Autodesk Inventor part; units mm, degrees
(part 2 of 2)
sketch "Sketch7" plane through (0, 0, 0) normal (0, -1, 0) x (1, 0, 0)
  line L0 (19.8255, 40.6005) -> (19.4339, 40.6005)
  line L1 (19.4339, 40.6005) -> (19.4339, 41.8395)
  line L2 (19.4339, 41.8395) -> (19.8255, 41.8395)
  line L3 (19.8255, 41.8395) -> (19.8255, 40.6005)
  line L4 (34.3949, 40.6005) -> (34.0033, 40.6005)
  line L5 (34.0033, 40.6005) -> (34.0033, 41.8395)
  line L6 (34.0033, 41.8395) -> (34.3949, 41.8395)
  line L7 (34.3949, 41.8395) -> (34.3949, 40.6005)
  line L8 (23.0894, 38.36) -> (23.0894, 38.66)
  line L9 (23.0894, 38.66) -> (23.7394, 38.66)
  line L10 (23.7394, 38.66) -> (23.7394, 38.36)
  line L11 (23.7394, 38.36) -> (23.0894, 38.36)
  line L12 (26.2394, 38.36) -> (25.5894, 38.36)
  line L13 (25.5894, 38.36) -> (25.5894, 38.66)
  line L14 (25.5894, 38.66) -> (26.2394, 38.66)
  line L15 (26.2394, 38.66) -> (26.2394, 38.36)
  line L16 (30.7394, 38.66) -> (30.7394, 38.36)
  line L17 (30.7394, 38.36) -> (30.0894, 38.36)
  line L18 (30.0894, 38.36) -> (30.0894, 38.66)
  line L19 (30.0894, 38.66) -> (30.7394, 38.66)
  line L20 (28.2394, 38.36) -> (27.5894, 38.36)
  line L21 (27.5894, 38.36) -> (27.5894, 38.66)
  line L22 (27.5894, 38.66) -> (28.2394, 38.66)
  line L23 (28.2394, 38.66) -> (28.2394, 38.36)
  line L24 (7.6945, 42.75) -> (6.6945, 42.75)
  line L25 (6.6945, 42.75) -> (6.6945, 43.25)
  line L26 (6.6945, 43.25) -> (7.6945, 43.25)
  line L27 (7.6945, 43.25) -> (7.6945, 42.75)
  line L28 (4.9445, 38.5) -> (4.9445, 37.5)
  line L29 (4.9445, 37.5) -> (4.4445, 37.5)
  line L30 (4.4445, 37.5) -> (4.4445, 38.5)
  line L31 (4.4445, 38.5) -> (4.9445, 38.5)
  line L32 (9.9445, 38.5) -> (9.9445, 37.5)
  line L33 (9.9445, 37.5) -> (9.4445, 37.5)
  line L34 (9.4445, 37.5) -> (9.4445, 38.5)
  line L35 (9.4445, 38.5) -> (9.9445, 38.5)
  line L36 (2.4445, 38.5) -> (2.4445, 37.5)
  line L37 (2.4445, 37.5) -> (1.9445, 37.5)
  line L38 (1.9445, 37.5) -> (1.9445, 38.5)
  line L39 (1.9445, 38.5) -> (2.4445, 38.5)
  line L40 (12.4445, 38.5) -> (12.4445, 37.5)
  line L41 (12.4445, 37.5) -> (11.9445, 37.5)
  line L42 (11.9445, 37.5) -> (11.9445, 38.5)
  line L43 (11.9445, 38.5) -> (12.4445, 38.5)
  line L44 (-20.3177, 45.8349) -> (-20.3177, 46.9651)
  line L45 (-20.3177, 46.9651) -> (-20.0677, 46.9651)
  line L46 (-20.0677, 46.9651) -> (-20.0677, 45.8349)
  line L47 (-20.0677, 45.8349) -> (-20.3177, 45.8349)
  line L48 (-5.2277, 42.75) -> (-5.2277, 42.5754)
  arc A0 (-8.0277, 42.5754) -> (-5.2277, 42.5754) centre (-6.6277, 43.35) ccw
  line L49 (-8.0277, 42.5754) -> (-8.0277, 43.2)
  line L50 (-8.0277, 43.2) -> (-7.3277, 43.2)
  line L51 (-7.3277, 43.2) -> (-7.3277, 42.75)
  line L52 (-7.3277, 42.75) -> (-5.2277, 42.75)
  line L53 (-5.2277, 44.1246) -> (-5.2277, 43.95)
  line L54 (-5.2277, 43.95) -> (-7.3277, 43.95)
  line L55 (-7.3277, 43.95) -> (-7.3277, 43.5)
  line L56 (-7.3277, 43.5) -> (-8.0277, 43.5)
  line L57 (-8.0277, 43.5) -> (-8.0277, 44.1246)
  arc A1 (-5.2277, 44.1246) -> (-8.0277, 44.1246) centre (-6.6277, 43.35) ccw
  arc A2 (-19.4577, 42.5754) -> (-16.6577, 42.5754) centre (-18.0577, 43.35) ccw
  line L58 (-19.4577, 42.5754) -> (-19.4577, 42.75)
  line L59 (-19.4577, 42.75) -> (-17.3577, 42.75)
  line L60 (-17.3577, 42.75) -> (-17.3577, 43.2)
  line L61 (-17.3577, 43.2) -> (-16.6577, 43.2)
  line L62 (-16.6577, 43.2) -> (-16.6577, 42.5754)
  arc A3 (-16.6577, 44.1246) -> (-19.4577, 44.1246) centre (-18.0577, 43.35) ccw
  line L63 (-16.6577, 44.1246) -> (-16.6577, 43.5)
  line L64 (-16.6577, 43.5) -> (-17.3577, 43.5)
  line L65 (-17.3577, 43.5) -> (-17.3577, 43.95)
  line L66 (-17.3577, 43.95) -> (-19.4577, 43.95)
  line L67 (-19.4577, 43.95) -> (-19.4577, 44.1246)
  arc A4 (-16.7877, 37.215) -> (-16.7877, 36.765) centre (-16.7877, 36.99) ccw
  arc A5 (-16.7877, 36.765) -> (-16.7877, 37.215) centre (-16.7877, 36.99) ccw
  arc A6 (-14.2477, 37.215) -> (-14.2477, 36.765) centre (-14.2477, 36.99) ccw
  arc A7 (-14.2477, 36.765) -> (-14.2477, 37.215) centre (-14.2477, 36.99) ccw
  arc A8 (-11.7077, 37.215) -> (-11.7077, 36.765) centre (-11.7077, 36.99) ccw
  arc A9 (-11.7077, 36.765) -> (-11.7077, 37.215) centre (-11.7077, 36.99) ccw
  arc A10 (-9.1677, 37.215) -> (-9.1677, 36.765) centre (-9.1677, 36.99) ccw
  arc A11 (-9.1677, 36.765) -> (-9.1677, 37.215) centre (-9.1677, 36.99) ccw
  arc A12 (-15.5177, 34.675) -> (-15.5177, 34.225) centre (-15.5177, 34.45) ccw
  arc A13 (-15.5177, 34.225) -> (-15.5177, 34.675) centre (-15.5177, 34.45) ccw
  arc A14 (-12.9777, 34.675) -> (-12.9777, 34.225) centre (-12.9777, 34.45) ccw
  arc A15 (-12.9777, 34.225) -> (-12.9777, 34.675) centre (-12.9777, 34.45) ccw
  arc A16 (-10.4377, 34.675) -> (-10.4377, 34.225) centre (-10.4377, 34.45) ccw
  arc A17 (-10.4377, 34.225) -> (-10.4377, 34.675) centre (-10.4377, 34.45) ccw
  arc A18 (-7.8977, 34.675) -> (-7.8977, 34.225) centre (-7.8977, 34.45) ccw
  arc A19 (-7.8977, 34.225) -> (-7.8977, 34.675) centre (-7.8977, 34.45) ccw
  line L68 (-4.6177, 45.8349) -> (-4.6177, 46.9651)
  line L69 (-4.6177, 46.9651) -> (-4.3677, 46.9651)
  line L70 (-4.3677, 46.9651) -> (-4.3677, 45.8349)
  line L71 (-4.3677, 45.8349) -> (-4.6177, 45.8349)
  line L72 (-30.7746, 41.22) -> (-30.7746, 41.78)
  arc A20 (-30.7746, 41.7814) -> (-30.7746, 41.78) centre (-30.5546, 41.78) ccw
  arc A21 (-30.5546, 42) -> (-30.7746, 41.7814) centre (-30.5546, 41.78) ccw
  line L73 (-30.5546, 42) -> (-29.9946, 42)
  arc A22 (-29.9919, 42) -> (-29.9946, 42) centre (-29.9946, 41.78) ccw
  arc A23 (-29.7746, 41.78) -> (-29.9919, 42) centre (-29.9946, 41.78) ccw
  line L74 (-29.7746, 41.78) -> (-29.7746, 41.22)
  arc A24 (-29.7746, 41.2186) -> (-29.7746, 41.22) centre (-29.9946, 41.22) ccw
  arc A25 (-29.9946, 41) -> (-29.7746, 41.2186) centre (-29.9946, 41.22) ccw
  line L75 (-29.9946, 41) -> (-30.5546, 41)
  arc A26 (-30.7746, 41.2186) -> (-30.5546, 41) centre (-30.5546, 41.22) ccw
  arc A27 (-30.7746, 41.22) -> (-30.7746, 41.2186) centre (-30.5546, 41.22) ccw
  line L76 (-25.7746, 41.22) -> (-25.7746, 41.78)
  arc A28 (-25.7746, 41.7814) -> (-25.7746, 41.78) centre (-25.5546, 41.78) ccw
  arc A29 (-25.5546, 42) -> (-25.7746, 41.7814) centre (-25.5546, 41.78) ccw
  line L77 (-25.5546, 42) -> (-24.9946, 42)
  arc A30 (-24.9919, 42) -> (-24.9946, 42) centre (-24.9946, 41.78) ccw
  arc A31 (-24.7746, 41.78) -> (-24.9919, 42) centre (-24.9946, 41.78) ccw
  line L78 (-24.7746, 41.78) -> (-24.7746, 41.22)
  arc A32 (-24.7746, 41.2186) -> (-24.7746, 41.22) centre (-24.9946, 41.22) ccw
  arc A33 (-24.9946, 41) -> (-24.7746, 41.2186) centre (-24.9946, 41.22) ccw
  line L79 (-24.9946, 41) -> (-25.5546, 41)
  arc A34 (-25.7746, 41.2186) -> (-25.5546, 41) centre (-25.5546, 41.22) ccw
  arc A35 (-25.7746, 41.22) -> (-25.7746, 41.2186) centre (-25.5546, 41.22) ccw
  line L80 (-33.125, 30.2845) -> (-32.455, 30.2845)
  line L81 (-32.455, 30.2845) -> (-32.455, 29.6145)
  line L82 (-32.455, 29.6145) -> (-33.125, 29.6145)
  line L83 (-33.125, 29.6145) -> (-33.125, 30.2845)
  line L84 (-33.125, 27.7445) -> (-32.455, 27.7445)
  line L85 (-32.455, 27.7445) -> (-32.455, 27.0745)
  line L86 (-32.455, 27.0745) -> (-33.125, 27.0745)
  line L87 (-33.125, 27.0745) -> (-33.125, 27.7445)
  circle A36 centre (31.5, -29) radius 2.1 projected
  circle A37 centre (-25.5, 29) radius 2.1 projected
  circle A38 centre (-25.5, -29) radius 2.1 projected
  circle A39 centre (31.5, 29) radius 2.1 projected
  arc A40 (40.5, -27.5) -> (36.5, -31.5) centre (40.5, -31.5) ccw projected
  line L88 (36.5, -31.5) -> (36.5, -44.5) projected
  arc A41 (33.5, -47.5) -> (36.5, -44.5) centre (33.5, -44.5) ccw projected
  line L89 (33.5, -47.5) -> (-33.5, -47.5) projected
  arc A42 (-36.5, -44.5) -> (-33.5, -47.5) centre (-33.5, -44.5) ccw projected
  line L90 (-36.5, -44.5) -> (-36.5, -31.5) projected
  arc A43 (-36.5, -31.5) -> (-40.5, -27.5) centre (-40.5, -31.5) ccw projected
  line L91 (-40.5, -27.5) -> (-44.5, -27.5) projected
  arc A44 (-47.5, -24.5) -> (-44.5, -27.5) centre (-44.5, -24.5) ccw projected
  line L92 (-47.5, -24.5) -> (-47.5, 24.5) projected
  arc A45 (-44.5, 27.5) -> (-47.5, 24.5) centre (-44.5, 24.5) ccw projected
  line L93 (-44.5, 27.5) -> (-40.5, 27.5) projected
  arc A46 (-40.5, 27.5) -> (-36.5, 31.5) centre (-40.5, 31.5) ccw projected
  line L94 (-36.5, 31.5) -> (-36.5, 44.5) projected
  arc A47 (-33.5, 47.5) -> (-36.5, 44.5) centre (-33.5, 44.5) ccw projected
  line L95 (-33.5, 47.5) -> (33.5, 47.5) projected
  arc A48 (36.5, 44.5) -> (33.5, 47.5) centre (33.5, 44.5) ccw projected
  line L96 (36.5, 44.5) -> (36.5, 31.5) projected
  arc A49 (36.5, 31.5) -> (40.5, 27.5) centre (40.5, 31.5) ccw projected
  line L97 (40.5, 27.5) -> (44.5, 27.5) projected
  arc A50 (47.5, 24.5) -> (44.5, 27.5) centre (44.5, 24.5) ccw projected
  line L98 (47.5, 24.5) -> (47.5, -24.5) projected
  arc A51 (44.5, -27.5) -> (47.5, -24.5) centre (44.5, -24.5) ccw projected
  line L99 (44.5, -27.5) -> (40.5, -27.5) projected
  circle A52 centre (40.395, 20.471) radius 1.5 projected
  circle A53 centre (-40.395, 20.471) radius 1.5 projected
  circle A54 centre (40.395, -20.471) radius 1.5 projected
  line L100 (43.9275, -13.9528) -> (44.5975, -13.9528)
  line L101 (44.5975, -13.9528) -> (44.5975, -14.6228)
  line L102 (44.5975, -14.6228) -> (43.9275, -14.6228)
  line L103 (43.9275, -14.6228) -> (43.9275, -13.9528)
  line L104 (43.9275, -11.4128) -> (44.5975, -11.4128)
  line L105 (44.5975, -11.4128) -> (44.5975, -12.0828)
  line L106 (44.5975, -12.0828) -> (43.9275, -12.0828)
  line L107 (43.9275, -12.0828) -> (43.9275, -11.4128)
  line L108 (43.9275, -8.8728) -> (44.5975, -8.8728)
  line L109 (44.5975, -8.8728) -> (44.5975, -9.5428)
  line L110 (44.5975, -9.5428) -> (43.9275, -9.5428)
  line L111 (43.9275, -9.5428) -> (43.9275, -8.8728)
  line L112 (43.9275, -6.3328) -> (44.5975, -6.3328)
  line L113 (44.5975, -6.3328) -> (44.5975, -7.0028)
  line L114 (44.5975, -7.0028) -> (43.9275, -7.0028)
  line L115 (43.9275, -7.0028) -> (43.9275, -6.3328)
  line L116 (43.9275, -3.7928) -> (44.5975, -3.7928)
  line L117 (44.5975, -3.7928) -> (44.5975, -4.4628)
  line L118 (44.5975, -4.4628) -> (43.9275, -4.4628)
  line L119 (43.9275, -4.4628) -> (43.9275, -3.7928)
  line L120 (43.9275, -1.2528) -> (44.5975, -1.2528)
  line L121 (44.5975, -1.2528) -> (44.5975, -1.9228)
  line L122 (44.5975, -1.9228) -> (43.9275, -1.9228)
  line L123 (43.9275, -1.9228) -> (43.9275, -1.2528)
  line L124 (43.9275, 1.2872) -> (44.5975, 1.2872)
  line L125 (44.5975, 1.2872) -> (44.5975, 0.6172)
  line L126 (44.5975, 0.6172) -> (43.9275, 0.6172)
  line L127 (43.9275, 0.6172) -> (43.9275, 1.2872)
  line L128 (43.9275, 3.8272) -> (44.5975, 3.8272)
  line L129 (44.5975, 3.8272) -> (44.5975, 3.1572)
  line L130 (44.5975, 3.1572) -> (43.9275, 3.1572)
  line L131 (43.9275, 3.1572) -> (43.9275, 3.8272)
  line L132 (43.9275, 6.3672) -> (44.5975, 6.3672)
  line L133 (44.5975, 6.3672) -> (44.5975, 5.6972)
  line L134 (44.5975, 5.6972) -> (43.9275, 5.6972)
  line L135 (43.9275, 5.6972) -> (43.9275, 6.3672)
  line L136 (43.9275, 8.9072) -> (44.5975, 8.9072)
  line L137 (44.5975, 8.9072) -> (44.5975, 8.2372)
  line L138 (44.5975, 8.2372) -> (43.9275, 8.2372)
  line L139 (43.9275, 8.2372) -> (43.9275, 8.9072)
  line L140 (43.9275, 11.4472) -> (44.5975, 11.4472)
  line L141 (44.5975, 11.4472) -> (44.5975, 10.7772)
  line L142 (44.5975, 10.7772) -> (43.9275, 10.7772)
  line L143 (43.9275, 10.7772) -> (43.9275, 11.4472)
  line L144 (43.9275, 13.9872) -> (44.5975, 13.9872)
  line L145 (44.5975, 13.9872) -> (44.5975, 13.3172)
  line L146 (44.5975, 13.3172) -> (43.9275, 13.3172)
  line L147 (43.9275, 13.3172) -> (43.9275, 13.9872)
  line L148 (-35.665, -22.7321) -> (-35.025, -22.7321)
  line L149 (-35.025, -22.7321) -> (-35.025, -23.3721)
  line L150 (-35.025, -23.3721) -> (-35.665, -23.3721)
  line L151 (-35.665, -23.3721) -> (-35.665, -22.7321)
  line L152 (-33.125, -22.7321) -> (-32.485, -22.7321)
  line L153 (-32.485, -22.7321) -> (-32.485, -23.3721)
  line L154 (-32.485, -23.3721) -> (-33.125, -23.3721)
  line L155 (-33.125, -23.3721) -> (-33.125, -22.7321)
  line L156 (-33.125, -20.1921) -> (-32.485, -20.1921)
  line L157 (-32.485, -20.1921) -> (-32.485, -20.8321)
  line L158 (-32.485, -20.8321) -> (-33.125, -20.8321)
  line L159 (-33.125, -20.8321) -> (-33.125, -20.1921)
  line L160 (-35.665, -20.1921) -> (-35.025, -20.1921)
  line L161 (-35.025, -20.1921) -> (-35.025, -20.8321)
  line L162 (-35.025, -20.8321) -> (-35.665, -20.8321)
  line L163 (-35.665, -20.8321) -> (-35.665, -20.1921)
  line L164 (-35.665, -17.6521) -> (-35.025, -17.6521)
  line L165 (-35.025, -17.6521) -> (-35.025, -18.2921)
  line L166 (-35.025, -18.2921) -> (-35.665, -18.2921)
  line L167 (-35.665, -18.2921) -> (-35.665, -17.6521)
  line L168 (-35.665, -15.1121) -> (-35.025, -15.1121)
  line L169 (-35.025, -15.1121) -> (-35.025, -15.7521)
  line L170 (-35.025, -15.7521) -> (-35.665, -15.7521)
  line L171 (-35.665, -15.7521) -> (-35.665, -15.1121)
  line L172 (-35.665, -12.5721) -> (-35.025, -12.5721)
  line L173 (-35.025, -12.5721) -> (-35.025, -13.2121)
  line L174 (-35.025, -13.2121) -> (-35.665, -13.2121)
  line L175 (-35.665, -13.2121) -> (-35.665, -12.5721)
  line L176 (-33.125, -12.5721) -> (-32.485, -12.5721)
  line L177 (-32.485, -12.5721) -> (-32.485, -13.2121)
  line L178 (-32.485, -13.2121) -> (-33.125, -13.2121)
  line L179 (-33.125, -13.2121) -> (-33.125, -12.5721)
  line L180 (-33.125, -15.1121) -> (-32.485, -15.1121)
  line L181 (-32.485, -15.1121) -> (-32.485, -15.7521)
  line L182 (-32.485, -15.7521) -> (-33.125, -15.7521)
  line L183 (-33.125, -15.7521) -> (-33.125, -15.1121)
  line L184 (-33.125, -17.6521) -> (-32.485, -17.6521)
  line L185 (-32.485, -17.6521) -> (-32.485, -18.2921)
  line L186 (-32.485, -18.2921) -> (-33.125, -18.2921)
  line L187 (-33.125, -18.2921) -> (-33.125, -17.6521)
  line L188 (-33.125, -5.2755) -> (-32.455, -5.2755)
  line L189 (-32.455, -5.2755) -> (-32.455, -5.9455)
  line L190 (-32.455, -5.9455) -> (-33.125, -5.9455)
  line L191 (-33.125, -5.9455) -> (-33.125, -5.2755)
  circle A55 centre (31.5, -29) radius 2.1 projected
  circle A56 centre (-25.5, 29) radius 2.1 projected
  circle A57 centre (-25.5, -29) radius 2.1 projected
  circle A58 centre (31.5, 29) radius 2.1 projected
  arc A59 (40.5, -27.5) -> (36.5, -31.5) centre (40.5, -31.5) ccw projected
  line L192 (36.5, -31.5) -> (36.5, -44.5) projected
  arc A60 (33.5, -47.5) -> (36.5, -44.5) centre (33.5, -44.5) ccw projected
  line L193 (33.5, -47.5) -> (-33.5, -47.5) projected
  arc A61 (-36.5, -44.5) -> (-33.5, -47.5) centre (-33.5, -44.5) ccw projected
  line L194 (-36.5, -44.5) -> (-36.5, -31.5) projected
  arc A62 (-36.5, -31.5) -> (-40.5, -27.5) centre (-40.5, -31.5) ccw projected
  line L195 (-40.5, -27.5) -> (-44.5, -27.5) projected
  arc A63 (-47.5, -24.5) -> (-44.5, -27.5) centre (-44.5, -24.5) ccw projected
  line L196 (-47.5, -24.5) -> (-47.5, 24.5) projected
  arc A64 (-44.5, 27.5) -> (-47.5, 24.5) centre (-44.5, 24.5) ccw projected
  line L197 (-44.5, 27.5) -> (-40.5, 27.5) projected
  arc A65 (-40.5, 27.5) -> (-36.5, 31.5) centre (-40.5, 31.5) ccw projected
  line L198 (-36.5, 31.5) -> (-36.5, 44.5) projected
  arc A66 (-33.5, 47.5) -> (-36.5, 44.5) centre (-33.5, 44.5) ccw projected
  line L199 (-33.5, 47.5) -> (33.5, 47.5) projected
  arc A67 (36.5, 44.5) -> (33.5, 47.5) centre (33.5, 44.5) ccw projected
  line L200 (36.5, 44.5) -> (36.5, 31.5) projected
  arc A68 (36.5, 31.5) -> (40.5, 27.5) centre (40.5, 31.5) ccw projected
  line L201 (40.5, 27.5) -> (44.5, 27.5) projected
  arc A69 (47.5, 24.5) -> (44.5, 27.5) centre (44.5, 24.5) ccw projected
  line L202 (47.5, 24.5) -> (47.5, -24.5) projected
  arc A70 (44.5, -27.5) -> (47.5, -24.5) centre (44.5, -24.5) ccw projected
  line L203 (44.5, -27.5) -> (40.5, -27.5) projected
  circle A71 centre (40.395, 20.471) radius 1.5 projected
  circle A72 centre (-40.395, 20.471) radius 1.5 projected
  circle A73 centre (40.395, -20.471) radius 1.5 projected
  line L204 (-33.125, -2.7355) -> (-32.455, -2.7355)
  line L205 (-32.455, -2.7355) -> (-32.455, -3.4055)
  line L206 (-32.455, -3.4055) -> (-33.125, -3.4055)
  line L207 (-33.125, -3.4055) -> (-33.125, -2.7355)
  line L208 (-33.125, -0.1955) -> (-32.455, -0.1955)
  line L209 (-32.455, -0.1955) -> (-32.455, -0.8655)
  line L210 (-32.455, -0.8655) -> (-33.125, -0.8655)
  line L211 (-33.125, -0.8655) -> (-33.125, -0.1955)
  line L212 (-33.125, 2.3445) -> (-32.455, 2.3445)
  line L213 (-32.455, 2.3445) -> (-32.455, 1.6745)
  line L214 (-32.455, 1.6745) -> (-33.125, 1.6745)
  line L215 (-33.125, 1.6745) -> (-33.125, 2.3445)
  line L216 (-35.665, 2.3445) -> (-34.995, 2.3445)
  line L217 (-34.995, 2.3445) -> (-34.995, 1.6745)
  line L218 (-34.995, 1.6745) -> (-35.665, 1.6745)
  line L219 (-35.665, 1.6745) -> (-35.665, 2.3445)
  circle A74 centre (31.5, -29) radius 2.1 projected
  circle A75 centre (-25.5, 29) radius 2.1 projected
  circle A76 centre (-25.5, -29) radius 2.1 projected
  circle A77 centre (31.5, 29) radius 2.1 projected
  arc A78 (40.5, -27.5) -> (36.5, -31.5) centre (40.5, -31.5) ccw projected
  line L220 (36.5, -31.5) -> (36.5, -44.5) projected
  arc A79 (33.5, -47.5) -> (36.5, -44.5) centre (33.5, -44.5) ccw projected
  line L221 (33.5, -47.5) -> (-33.5, -47.5) projected
  arc A80 (-36.5, -44.5) -> (-33.5, -47.5) centre (-33.5, -44.5) ccw projected
  line L222 (-36.5, -44.5) -> (-36.5, -31.5) projected
  arc A81 (-36.5, -31.5) -> (-40.5, -27.5) centre (-40.5, -31.5) ccw projected
  line L223 (-40.5, -27.5) -> (-44.5, -27.5) projected
  arc A82 (-47.5, -24.5) -> (-44.5, -27.5) centre (-44.5, -24.5) ccw projected
  line L224 (-47.5, -24.5) -> (-47.5, 24.5) projected
  arc A83 (-44.5, 27.5) -> (-47.5, 24.5) centre (-44.5, 24.5) ccw projected
  line L225 (-44.5, 27.5) -> (-40.5, 27.5) projected
  arc A84 (-40.5, 27.5) -> (-36.5, 31.5) centre (-40.5, 31.5) ccw projected
  line L226 (-36.5, 31.5) -> (-36.5, 44.5) projected
  arc A85 (-33.5, 47.5) -> (-36.5, 44.5) centre (-33.5, 44.5) ccw projected
  line L227 (-33.5, 47.5) -> (33.5, 47.5) projected
  arc A86 (36.5, 44.5) -> (33.5, 47.5) centre (33.5, 44.5) ccw projected
  line L228 (36.5, 44.5) -> (36.5, 31.5) projected
  arc A87 (36.5, 31.5) -> (40.5, 27.5) centre (40.5, 31.5) ccw projected
  line L229 (40.5, 27.5) -> (44.5, 27.5) projected
  arc A88 (47.5, 24.5) -> (44.5, 27.5) centre (44.5, 24.5) ccw projected
  line L230 (47.5, 24.5) -> (47.5, -24.5) projected
  arc A89 (44.5, -27.5) -> (47.5, -24.5) centre (44.5, -24.5) ccw projected
  line L231 (44.5, -27.5) -> (40.5, -27.5) projected
  circle A90 centre (40.395, 20.471) radius 1.5 projected
  circle A91 centre (-40.395, 20.471) radius 1.5 projected
  circle A92 centre (40.395, -20.471) radius 1.5 projected
  line L232 (-35.665, -0.1955) -> (-34.995, -0.1955)
  line L233 (-34.995, -0.1955) -> (-34.995, -0.8655)
  line L234 (-34.995, -0.8655) -> (-35.665, -0.8655)
  line L235 (-35.665, -0.8655) -> (-35.665, -0.1955)
  line L236 (-35.665, -2.7355) -> (-34.995, -2.7355)
  line L237 (-34.995, -2.7355) -> (-34.995, -3.4055)
  line L238 (-34.995, -3.4055) -> (-35.665, -3.4055)
  line L239 (-35.665, -3.4055) -> (-35.665, -2.7355)
  line L240 (-35.665, -5.2755) -> (-34.995, -5.2755)
  line L241 (-34.995, -5.2755) -> (-34.995, -5.9455)
  line L242 (-34.995, -5.9455) -> (-35.665, -5.9455)
  line L243 (-35.665, -5.9455) -> (-35.665, -5.2755)
  line L244 (-33.125, 9.9645) -> (-32.455, 9.9645)
  line L245 (-32.455, 9.9645) -> (-32.455, 9.2945)
  line L246 (-32.455, 9.2945) -> (-33.125, 9.2945)
  line L247 (-33.125, 9.2945) -> (-33.125, 9.9645)
  line L248 (-33.125, 7.4245) -> (-32.455, 7.4245)
  line L249 (-32.455, 7.4245) -> (-32.455, 6.7545)
  line L250 (-32.455, 6.7545) -> (-33.125, 6.7545)
  line L251 (-33.125, 6.7545) -> (-33.125, 7.4245)
  line L252 (-33.125, 4.8845) -> (-32.455, 4.8845)
  line L253 (-32.455, 4.8845) -> (-32.455, 4.2145)
  line L254 (-32.455, 4.2145) -> (-33.125, 4.2145)
  line L255 (-33.125, 4.2145) -> (-33.125, 4.8845)
  circle A93 centre (31.5, -29) radius 2.1 projected
  circle A94 centre (-25.5, 29) radius 2.1 projected
  circle A95 centre (-25.5, -29) radius 2.1 projected
  circle A96 centre (31.5, 29) radius 2.1 projected
  arc A97 (40.5, -27.5) -> (36.5, -31.5) centre (40.5, -31.5) ccw projected
  line L256 (36.5, -31.5) -> (36.5, -44.5) projected
  arc A98 (33.5, -47.5) -> (36.5, -44.5) centre (33.5, -44.5) ccw projected
  line L257 (33.5, -47.5) -> (-33.5, -47.5) projected
  arc A99 (-36.5, -44.5) -> (-33.5, -47.5) centre (-33.5, -44.5) ccw projected
  line L258 (-36.5, -44.5) -> (-36.5, -31.5) projected
  arc A100 (-36.5, -31.5) -> (-40.5, -27.5) centre (-40.5, -31.5) ccw projected
  line L259 (-40.5, -27.5) -> (-44.5, -27.5) projected
  arc A101 (-47.5, -24.5) -> (-44.5, -27.5) centre (-44.5, -24.5) ccw projected
  line L260 (-47.5, -24.5) -> (-47.5, 24.5) projected
  arc A102 (-44.5, 27.5) -> (-47.5, 24.5) centre (-44.5, 24.5) ccw projected
  line L261 (-44.5, 27.5) -> (-40.5, 27.5) projected
  arc A103 (-40.5, 27.5) -> (-36.5, 31.5) centre (-40.5, 31.5) ccw projected
  line L262 (-36.5, 31.5) -> (-36.5, 44.5) projected
  arc A104 (-33.5, 47.5) -> (-36.5, 44.5) centre (-33.5, 44.5) ccw projected
  line L263 (-33.5, 47.5) -> (33.5, 47.5) projected
  arc A105 (36.5, 44.5) -> (33.5, 47.5) centre (33.5, 44.5) ccw projected
  line L264 (36.5, 44.5) -> (36.5, 31.5) projected
  arc A106 (36.5, 31.5) -> (40.5, 27.5) centre (40.5, 31.5) ccw projected
  line L265 (40.5, 27.5) -> (44.5, 27.5) projected
  arc A107 (47.5, 24.5) -> (44.5, 27.5) centre (44.5, 24.5) ccw projected
  line L266 (47.5, 24.5) -> (47.5, -24.5) projected
  arc A108 (44.5, -27.5) -> (47.5, -24.5) centre (44.5, -24.5) ccw projected
  line L267 (44.5, -27.5) -> (40.5, -27.5) projected
  circle A109 centre (40.395, 20.471) radius 1.5 projected
  circle A110 centre (-40.395, 20.471) radius 1.5 projected
  circle A111 centre (40.395, -20.471) radius 1.5 projected
  line L268 (-35.665, 4.8845) -> (-34.995, 4.8845)
  line L269 (-34.995, 4.8845) -> (-34.995, 4.2145)
  line L270 (-34.995, 4.2145) -> (-35.665, 4.2145)
  line L271 (-35.665, 4.2145) -> (-35.665, 4.8845)
  line L272 (-35.665, 7.4245) -> (-34.995, 7.4245)
  line L273 (-34.995, 7.4245) -> (-34.995, 6.7545)
  line L274 (-34.995, 6.7545) -> (-35.665, 6.7545)
  line L275 (-35.665, 6.7545) -> (-35.665, 7.4245)
  circle A112 centre (31.5, -29) radius 2.1 projected
  circle A113 centre (-25.5, 29) radius 2.1 projected
  circle A114 centre (-25.5, -29) radius 2.1 projected
  circle A115 centre (31.5, 29) radius 2.1 projected
  arc A116 (40.5, -27.5) -> (36.5, -31.5) centre (40.5, -31.5) ccw projected
  line L276 (36.5, -31.5) -> (36.5, -44.5) projected
  arc A117 (33.5, -47.5) -> (36.5, -44.5) centre (33.5, -44.5) ccw projected
  line L277 (33.5, -47.5) -> (-33.5, -47.5) projected
  arc A118 (-36.5, -44.5) -> (-33.5, -47.5) centre (-33.5, -44.5) ccw projected
  line L278 (-36.5, -44.5) -> (-36.5, -31.5) projected
  arc A119 (-36.5, -31.5) -> (-40.5, -27.5) centre (-40.5, -31.5) ccw projected
  line L279 (-40.5, -27.5) -> (-44.5, -27.5) projected
  arc A120 (-47.5, -24.5) -> (-44.5, -27.5) centre (-44.5, -24.5) ccw projected
  line L280 (-47.5, -24.5) -> (-47.5, 24.5) projected
  arc A121 (-44.5, 27.5) -> (-47.5, 24.5) centre (-44.5, 24.5) ccw projected
  line L281 (-44.5, 27.5) -> (-40.5, 27.5) projected
  arc A122 (-40.5, 27.5) -> (-36.5, 31.5) centre (-40.5, 31.5) ccw projected
  line L282 (-36.5, 31.5) -> (-36.5, 44.5) projected
  arc A123 (-33.5, 47.5) -> (-36.5, 44.5) centre (-33.5, 44.5) ccw projected
  line L283 (-33.5, 47.5) -> (33.5, 47.5) projected
  arc A124 (36.5, 44.5) -> (33.5, 47.5) centre (33.5, 44.5) ccw projected
  line L284 (36.5, 44.5) -> (36.5, 31.5) projected
  arc A125 (36.5, 31.5) -> (40.5, 27.5) centre (40.5, 31.5) ccw projected
  line L285 (40.5, 27.5) -> (44.5, 27.5) projected
  arc A126 (47.5, 24.5) -> (44.5, 27.5) centre (44.5, 24.5) ccw projected
  line L286 (47.5, 24.5) -> (47.5, -24.5) projected
  arc A127 (44.5, -27.5) -> (47.5, -24.5) centre (44.5, -24.5) ccw projected
  line L287 (44.5, -27.5) -> (40.5, -27.5) projected
  circle A128 centre (40.395, 20.471) radius 1.5 projected
  circle A129 centre (-40.395, 20.471) radius 1.5 projected
  circle A130 centre (40.395, -20.471) radius 1.5 projected
  line L288 (-35.665, 9.9645) -> (-34.995, 9.9645)
  line L289 (-34.995, 9.9645) -> (-34.995, 9.2945)
  line L290 (-34.995, 9.2945) -> (-35.665, 9.2945)
  line L291 (-35.665, 9.2945) -> (-35.665, 9.9645)
  line L292 (-35.665, 12.5045) -> (-34.995, 12.5045)
  line L293 (-34.995, 12.5045) -> (-34.995, 11.8345)
  line L294 (-34.995, 11.8345) -> (-35.665, 11.8345)
  line L295 (-35.665, 11.8345) -> (-35.665, 12.5045)
  line L296 (-35.665, 15.0445) -> (-34.995, 15.0445)
  line L297 (-34.995, 15.0445) -> (-34.995, 14.3745)
  line L298 (-34.995, 14.3745) -> (-35.665, 14.3745)
  line L299 (-35.665, 14.3745) -> (-35.665, 15.0445)
  line L300 (-35.665, 17.5845) -> (-34.995, 17.5845)
  line L301 (-34.995, 17.5845) -> (-34.995, 16.9145)
  line L302 (-34.995, 16.9145) -> (-35.665, 16.9145)
  line L303 (-35.665, 16.9145) -> (-35.665, 17.5845)
  line L304 (-35.665, 20.1245) -> (-34.995, 20.1245)
  line L305 (-34.995, 20.1245) -> (-34.995, 19.4545)
  line L306 (-34.995, 19.4545) -> (-35.665, 19.4545)
  line L307 (-35.665, 19.4545) -> (-35.665, 20.1245)
  line L308 (-35.665, 22.6645) -> (-34.995, 22.6645)
  line L309 (-34.995, 22.6645) -> (-34.995, 21.9945)
  line L310 (-34.995, 21.9945) -> (-35.665, 21.9945)
  line L311 (-35.665, 21.9945) -> (-35.665, 22.6645)
  line L312 (-33.125, 22.6645) -> (-32.455, 22.6645)
  line L313 (-32.455, 22.6645) -> (-32.455, 21.9945)
  line L314 (-32.455, 21.9945) -> (-33.125, 21.9945)
  line L315 (-33.125, 21.9945) -> (-33.125, 22.6645)
  line L316 (-33.125, 20.1245) -> (-32.455, 20.1245)
  line L317 (-32.455, 20.1245) -> (-32.455, 19.4545)
  line L318 (-32.455, 19.4545) -> (-33.125, 19.4545)
  line L319 (-33.125, 19.4545) -> (-33.125, 20.1245)
  line L320 (-33.125, 17.5845) -> (-32.455, 17.5845)
  line L321 (-32.455, 17.5845) -> (-32.455, 16.9145)
  line L322 (-32.455, 16.9145) -> (-33.125, 16.9145)
  line L323 (-33.125, 16.9145) -> (-33.125, 17.5845)
  line L324 (-33.125, 15.0445) -> (-32.455, 15.0445)
  line L325 (-32.455, 15.0445) -> (-32.455, 14.3745)
  line L326 (-32.455, 14.3745) -> (-33.125, 14.3745)
  line L327 (-33.125, 14.3745) -> (-33.125, 15.0445)
  line L328 (-33.125, 12.5045) -> (-32.455, 12.5045)
  line L329 (-32.455, 12.5045) -> (-32.455, 11.8345)
  line L330 (-32.455, 11.8345) -> (-33.125, 11.8345)
  line L331 (-33.125, 11.8345) -> (-33.125, 12.5045)
  line L332 (-33.125, 25.2045) -> (-32.455, 25.2045)
  line L333 (-32.455, 25.2045) -> (-32.455, 24.5345)
  line L334 (-32.455, 24.5345) -> (-33.125, 24.5345)
  line L335 (-33.125, 24.5345) -> (-33.125, 25.2045)
  line L336 (-35.665, 25.2045) -> (-34.995, 25.2045)
  line L337 (-34.995, 25.2045) -> (-34.995, 24.5345)
  line L338 (-34.995, 24.5345) -> (-35.665, 24.5345)
  line L339 (-35.665, 24.5345) -> (-35.665, 25.2045)
  line L340 (-35.665, 27.7445) -> (-34.995, 27.7445)
  line L341 (-34.995, 27.7445) -> (-34.995, 27.0745)
  line L342 (-34.995, 27.0745) -> (-35.665, 27.0745)
  line L343 (-35.665, 27.0745) -> (-35.665, 27.7445)
  line L344 (-35.665, 30.2845) -> (-34.995, 30.2845)
  line L345 (-34.995, 30.2845) -> (-34.995, 29.6145)
  line L346 (-34.995, 29.6145) -> (-35.665, 29.6145)
  line L347 (-35.665, 29.6145) -> (-35.665, 30.2845)
  line L348 (-1.4612, 46.33) -> (-1.4612, 45.63)
  line L349 (-1.4612, 45.63) -> (-1.8612, 45.63)
  line L350 (-1.8612, 45.63) -> (-1.8612, 46.33)
  line L351 (-1.8612, 46.33) -> (-1.4612, 46.33)
  line L352 (-1.4612, 43.79) -> (-1.4612, 43.09)
  line L353 (-1.4612, 43.09) -> (-1.8612, 43.09)
  line L354 (-1.8612, 43.09) -> (-1.8612, 43.79)
  line L355 (-1.8612, 43.79) -> (-1.4612, 43.79)
  line L356 (-1.4612, 41.25) -> (-1.4612, 40.55)
  line L357 (-1.4612, 40.55) -> (-1.8612, 40.55)
  line L358 (-1.8612, 40.55) -> (-1.8612, 41.25)
  line L359 (-1.8612, 41.25) -> (-1.4612, 41.25)
  line L360 (-1.4612, 38.71) -> (-1.4612, 38.01)
  line L361 (-1.4612, 38.01) -> (-1.8612, 38.01)
  line L362 (-1.8612, 38.01) -> (-1.8612, 38.71)
  line L363 (-1.8612, 38.71) -> (-1.4612, 38.71)
  line L364 (-1.4612, 36.17) -> (-1.4612, 35.47)
  line L365 (-1.4612, 35.47) -> (-1.8612, 35.47)
  line L366 (-1.8612, 35.47) -> (-1.8612, 36.17)
  line L367 (-1.8612, 36.17) -> (-1.4612, 36.17)
  circle A131 centre (31.5, -29) radius 2.1 projected
  circle A132 centre (-25.5, 29) radius 2.1 projected
  circle A133 centre (-25.5, -29) radius 2.1 projected
  circle A134 centre (31.5, 29) radius 2.1 projected
  arc A135 (40.5, -27.5) -> (36.5, -31.5) centre (40.5, -31.5) ccw projected
  line L368 (36.5, -31.5) -> (36.5, -44.5) projected
  arc A136 (33.5, -47.5) -> (36.5, -44.5) centre (33.5, -44.5) ccw projected
  line L369 (33.5, -47.5) -> (-33.5, -47.5) projected
  arc A137 (-36.5, -44.5) -> (-33.5, -47.5) centre (-33.5, -44.5) ccw projected
  line L370 (-36.5, -44.5) -> (-36.5, -31.5) projected
  arc A138 (-36.5, -31.5) -> (-40.5, -27.5) centre (-40.5, -31.5) ccw projected
  line L371 (-40.5, -27.5) -> (-44.5, -27.5) projected
  arc A139 (-47.5, -24.5) -> (-44.5, -27.5) centre (-44.5, -24.5) ccw projected
  line L372 (-47.5, -24.5) -> (-47.5, 24.5) projected
  arc A140 (-44.5, 27.5) -> (-47.5, 24.5) centre (-44.5, 24.5) ccw projected
  line L373 (-44.5, 27.5) -> (-40.5, 27.5) projected
  arc A141 (-40.5, 27.5) -> (-36.5, 31.5) centre (-40.5, 31.5) ccw projected
  line L374 (-36.5, 31.5) -> (-36.5, 44.5) projected
  arc A142 (-33.5, 47.5) -> (-36.5, 44.5) centre (-33.5, 44.5) ccw projected
  line L375 (-33.5, 47.5) -> (33.5, 47.5) projected
  arc A143 (36.5, 44.5) -> (33.5, 47.5) centre (33.5, 44.5) ccw projected
  line L376 (36.5, 44.5) -> (36.5, 31.5) projected
  arc A144 (36.5, 31.5) -> (40.5, 27.5) centre (40.5, 31.5) ccw projected
  line L377 (40.5, 27.5) -> (44.5, 27.5) projected
  arc A145 (47.5, 24.5) -> (44.5, 27.5) centre (44.5, 24.5) ccw projected
  line L378 (47.5, 24.5) -> (47.5, -24.5) projected
  arc A146 (44.5, -27.5) -> (47.5, -24.5) centre (44.5, -24.5) ccw projected
  line L379 (44.5, -27.5) -> (40.5, -27.5) projected
  circle A147 centre (40.395, 20.471) radius 1.5 projected
  circle A148 centre (-40.395, 20.471) radius 1.5 projected
  circle A149 centre (40.395, -20.471) radius 1.5 projected
  line L380 (-1.4612, 33.63) -> (-1.4612, 32.93)
  line L381 (-1.4612, 32.93) -> (-1.8612, 32.93)
  line L382 (-1.8612, 32.93) -> (-1.8612, 33.63)
  line L383 (-1.8612, 33.63) -> (-1.4612, 33.63)
  line L384 (-1.4612, 31.09) -> (-1.4612, 30.39)
  line L385 (-1.4612, 30.39) -> (-1.8612, 30.39)
  line L386 (-1.8612, 30.39) -> (-1.8612, 31.09)
  line L387 (-1.8612, 31.09) -> (-1.4612, 31.09)
  line L388 (-1.4612, 28.55) -> (-1.4612, 27.85)
  line L389 (-1.4612, 27.85) -> (-1.8612, 27.85)
  line L390 (-1.8612, 27.85) -> (-1.8612, 28.55)
  line L391 (-1.8612, 28.55) -> (-1.4612, 28.55)
  line L392 (16.5728, 28.55) -> (16.5728, 27.85)
  line L393 (16.5728, 27.85) -> (16.1728, 27.85)
  line L394 (16.1728, 27.85) -> (16.1728, 28.55)
  line L395 (16.1728, 28.55) -> (16.5728, 28.55)
  line L396 (16.5728, 31.09) -> (16.5728, 30.39)
  line L397 (16.5728, 30.39) -> (16.1728, 30.39)
  line L398 (16.1728, 30.39) -> (16.1728, 31.09)
  line L399 (16.1728, 31.09) -> (16.5728, 31.09)
  line L400 (16.5728, 33.63) -> (16.5728, 32.93)
  line L401 (16.5728, 32.93) -> (16.1728, 32.93)
  line L402 (16.1728, 32.93) -> (16.1728, 33.63)
  line L403 (16.1728, 33.63) -> (16.5728, 33.63)
  line L404 (16.5728, 36.17) -> (16.5728, 35.47)
  line L405 (16.5728, 35.47) -> (16.1728, 35.47)
  line L406 (16.1728, 35.47) -> (16.1728, 36.17)
  line L407 (16.1728, 36.17) -> (16.5728, 36.17)
  line L408 (16.5728, 38.71) -> (16.5728, 38.01)
  line L409 (16.5728, 38.01) -> (16.1728, 38.01)
  line L410 (16.1728, 38.01) -> (16.1728, 38.71)
  line L411 (16.1728, 38.71) -> (16.5728, 38.71)
  line L412 (16.5728, 41.25) -> (16.5728, 40.55)
  line L413 (16.5728, 40.55) -> (16.1728, 40.55)
  line L414 (16.1728, 40.55) -> (16.1728, 41.25)
  line L415 (16.1728, 41.25) -> (16.5728, 41.25)
  line L416 (16.5728, 43.79) -> (16.5728, 43.09)
  line L417 (16.5728, 43.09) -> (16.1728, 43.09)
  line L418 (16.1728, 43.09) -> (16.1728, 43.79)
  line L419 (16.1728, 43.79) -> (16.5728, 43.79)
  line L420 (16.5728, 46.33) -> (16.5728, 45.63)
  line L421 (16.5728, 45.63) -> (16.1728, 45.63)
  line L422 (16.1728, 45.63) -> (16.1728, 46.33)
  line L423 (16.1728, 46.33) -> (16.5728, 46.33)
  point P0 (0, 0)
  constraints: 704 end point, 178 vertical, 174 horizontal, 72 point on circle, 36 centre point, 460 other
extrude "Extrusion3" cut sketch "Sketch7" against normal blind 10 contours L0 L1 L2 L3 | L4 L5 L6 L7 | L8 L9 L10 L11 | L12 L13 L14 L15 | L16 L17 L18 L19 | L20 L21 L22 L23 | L24 L25 L26 L27 | L28 L29 L30 L31 | L32 L33 L34 L35 | L36 L37 L38 L39 | L40 L41 L42 L43 | L44 L45 L46 L47 | L48 A0 L49 L50 L51 L52 | L53 L54 L55 L56 L57 A1 | L58 L59 L60 L61 L62 A2 | L63 L64 L65 L66 L67 A3 | A5 A4 | A7 A6 | A9 A8 | A11 A10 | A13 A12 | A15 A14 | A17 A16 | A19 A18 | L68 L69 L70 L71 | A27 A26 | L72 A20 L73 A22 A23 L74 A24 L75 A27 | A20 | A24 | A35 A34 | L76 A28 L77 A30 A31 L78 A32 L79 A35 | A28 | A32 | L80 L81 L82 L83 | L84 L85 L86 L87 | A36 | A37 | A38 | A39 | A52 | A53 | A54 | L100 L101 L102 L103 | L104 L105 L106 L107 | L108 L109 L110 L111 | L112 L113 L114 L115 | L116 L117 L118 L119 | L120 L121 L122 L123 | L124 L125 L126 L127 | L128 L129 L130 L131 | L132 L133 L134 L135 | L136 L137 L138 L139 | L140 L141 L142 L143 | L144 L145 L146 L147 | L148 L149 L150 L151 | L152 L153 L154 L155 | L156 L157 L158 L159 | L160 L161 L162 L163 | L164 L165 L166 L167 | L168 L169 L170 L171 | L172 L173 L174 L175 | L176 L177 L178 L179 | L180 L181 L182 L183 | L184 L185 L186 L187 | L188 L189 L190 L191 | L204 L205 L206 L207 | L208 L209 L210 L211 | L212 L213 L214 L215 | L216 L217 L218 L219 | L232 L233 L234 L235 | L236 L237 L238 L239 | L240 L241 L242 L243 | L244 L245 L246 L247 | L248 L249 L250 L251 | L252 L253 L254 L255 | L268 L269 L270 L271 | L272 L273 L274 L275 | L288 L289 L290 L291 | L292 L293 L294 L295 | L296 L297 L298 L299 | L300 L301 L302 L303 | L304 L305 L306 L307 | L308 L309 L310 L311 | L312 L313 L314 L315 | L316 L317 L318 L319 | L320 L321 L322 L323 | L324 L325 L326 L327 | L328 L329 L330 L331 | L332 L333 L334 L335 | L336 L337 L338 L339 | L340 L341 L342 L343 | L344 L345 L346 L347 | L348 L349 L350 L351 | L352 L353 L354 L355 | L356 L357 L358 L359 | L360 L361 L362 L363 | L364 L365 L366 L367 | L380 L381 L382 L383 | L384 L385 L386 L387 | L388 L389 L390 L391 | L392 L393 L394 L395 | L396 L397 L398 L399 | L400 L401 L402 L403 | L404 L405 L406 L407 | L408 L409 L410 L411 | L412 L413 L414 L415 | L416 L417 L418 L419 | L420 L421 L422 L423
equation "\"d19\" = d21"
equation "\"d22\" = d18"
equation "\"d23\" = d18"
equation "\"d24\" = d19"
equation "\"d25\" = d18"
equation "\"d26\" = d21"
body "Solid1"
